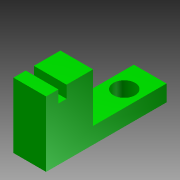
# Autodesk Inventor part: grip2
Saved by Autodesk Inventor 2015 SP1 (Build 190203100, 203)
## iProperties
Created: 2011-06-13
Part Number: grip2
Document SubType Name: Modeling
Designer: ijs09
Density: 1 g/cm^3
Material: Generic
Appearance: Default
Author: ijs09
Autodesk Inventor part; units mm, degrees
ref_plane "YZ Plane" through (0, 0, 0) normal (1, 0, 0) x (0, 1, 0)
ref_plane "XZ Plane" through (0, 0, 0) normal (0, 1, 0) x (-1, 0, 0)
ref_plane "XY Plane" through (0, 0, 0) normal (0, 0, 1) x (1, 0, 0)
sketch "Sketch2" plane through (0, 0, 0) normal (1, 0, 0) x (0, 1, 0)
  line L0 (-8.2312, 6.508) -> (-8.2312, 3.508)
  line L1 (-8.2312, 3.508) -> (-10.2312, 3.508)
  line L2 (-10.2312, 3.508) -> (-10.2312, 6.508)
  line L3 (-10.2312, 6.508) -> (-13.2312, 6.508)
  line L4 (-13.2312, 6.508) -> (-13.2312, -9.492)
  line L5 (-13.2312, -9.492) -> (16.2688, -9.492)
  line L6 (16.2688, -5.492) -> (-1.7312, -5.492)
  line L7 (-1.7312, -5.492) -> (-1.7312, 6.508)
  line L8 (16.2688, -9.492) -> (16.2688, -5.492)
  line L9 (-1.7312, 6.508) -> (-8.2312, 6.508)
  point P0 (0, 0)
  dimension "d2" = 2
  dimension "d3" = 3
  dimension "d4" = 16
  dimension "d9" = 12
  dimension "d10" = 29.5
  dimension "d11" = 24.5
  dimension "d12" = 18
  dimension "d22" = 4
  constraints: 20 end point, 2 parallel, 1 perpendicular
  measures "d2" distance between parallel lines of L2 L0
  measures "d3" distance between parallel lines of L1 L3
  measures "d4" distance between parallel lines of L5 L3
  measures "d9" distance between parallel lines of L9 L6
  measures "d10" distance between parallel lines of L8 L4
  measures "d11" distance between parallel lines of L0 L8
  measures "d12" distance between parallel lines of L8 L7
  measures "d22" distance of L5.end L6.start
extrude "Extrusion1" add sketch "Sketch2" along normal blind 8
sketch "Sketch3" plane through (0, -1.7312, -5.492) normal (0, 0, 1) x (1, 0, 0)
  line L0 (0, 18) -> (8, 18) projected
  line L1 (0, 0) -> (0, 18) projected
  point P0 (0, 1.7312)
  point P1 (4, 11.65)
  dimension "d13" = 6.35
  dimension "d14" = 4
  measures "d13" distance from line of L0 point (4, 11.65)
  measures "d14" distance from line of L1 point (4, 11.65)
hole "Hole1" at (4, 9.9188, -5.492) direction (0, 0, -1) diameter 5.3 depth 8 tip angle 118
body "Solid1"
